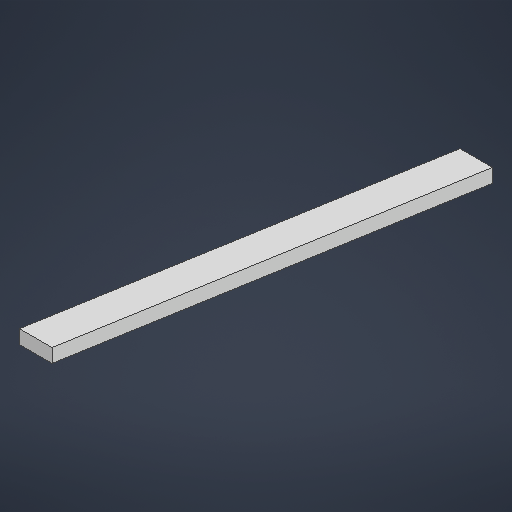
# Autodesk Inventor part: S_2x4x48.76
Saved by Autodesk Inventor 2027.1 (Build 311270010, 270A)
## iProperties
Created: 2026-09-01
Part Number: S_2x4x48.76
Material: Generic
Document SubType Name: Modeling
Designer: jorda
Density: 1 g/cm^3
Appearance: Default
Author: jorda
Autodesk Inventor part; units mm, degrees
ref_plane "YZ Plane" through (0, 0, 0) normal (1, 0, 0) x (0, 1, 0)
ref_plane "XZ Plane" through (0, 0, 0) normal (0, 1, 0) x (-1, 0, 0)
ref_plane "XY Plane" through (0, 0, 0) normal (0, 0, 1) x (1, 0, 0)
sketch "Sketch1" plane through (0, 0, 0) normal (0, 1, 0) x (-1, 0, 0)
  line L0 (214.6102, -0.0199) -> (304.9164, -0.0199)
  line L1 (304.9164, -0.0199) -> (214.6102, -0.0199)
  line L2 (304.9164, -0.0199) -> (127, -1041.4)
  line L3 (127, -1041.4) -> (38.2671, -1041.4)
  line L4 (39.368, -1026.4384) -> (214.6102, -0.0199)
  line L5 (38.2671, -1041.4) -> (36.8136, -1041.4)
  line L6 (39.368, -1026.4384) -> (36.8136, -1041.4)
  point P0 (0, 0)
  constraints: 14 end point, 4 horizontal
extrude "Extrusion1" add sketch "Sketch1" along normal blind 38.1
body "Solid1"
